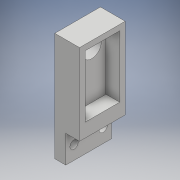
# Autodesk Inventor part: armpart2
Saved by Autodesk Inventor 2018.3 (Build 223284000, 284)
## iProperties
Created: 2019-11-01
Part Number: armpart2
Material: 一般
Document SubType Name: Modeling
Designer: Eiji Nishizawa
Density: 1 g/cm^3
Appearance: 既定
Mass: 3.44311 g
Surface Area: 26.3012 cm^2
Volume: 3.44311 cm^3
Author: Eiji Nishizawa
Autodesk Inventor part; units mm, degrees
ref_plane "YZ Plane" through (0, 0, 0) normal (1, 0, 0) x (0, 1, 0)
ref_plane "XZ Plane" through (0, 0, 0) normal (0, 1, 0) x (-1, 0, 0)
ref_plane "XY Plane" through (0, 0, 0) normal (0, 0, 1) x (1, 0, 0)
sketch "スケッチ1" plane through (0, 0, 0) normal (1, 0, 0) x (0, 1, 0)
  line L0 (8.6678, 22.4898) -> (-7.9322, 22.4898)
  line L1 (-7.9322, 22.4898) -> (-7.9322, -15.0102)
  line L2 (-7.9322, -15.0102) -> (8.6678, -15.0102)
  line L3 (8.6678, -15.0102) -> (8.6678, 22.4898)
  line L4 (8.6678, 22.4898) -> (6.6678, 22.4898)
  line L5 (6.6678, 22.4898) -> (6.6678, -0.0102)
  line L6 (6.6678, -0.0102) -> (8.6678, -0.0102)
  line L7 (8.6678, -0.0102) -> (8.6678, 22.4898)
  line L8 (-7.9322, 22.4898) -> (-5.9322, 22.4898)
  line L9 (-5.9322, 22.4898) -> (-5.9322, -0.0102)
  line L10 (-5.9322, -0.0102) -> (-7.9322, -0.0102)
  line L11 (-7.9322, -0.0102) -> (-7.9322, 22.4898)
  line L12 (8.6678, 22.4898) -> (-7.9322, 22.4898)
  line L13 (-7.9322, 22.4898) -> (-7.9322, 24.4898)
  line L14 (-7.9322, 24.4898) -> (8.6678, 24.4898)
  line L15 (8.6678, 24.4898) -> (8.6678, 22.4898)
  circle A0 centre (5.6678, -10.0102) radius 1.5
  circle A1 centre (-4.9322, -10.0102) radius 1.5
  point P0 (0, 0)
  dimension "d1" = 2
  dimension "d2" = 2
  dimension "d3" = 15
  dimension "d4" = 22.5
  dimension "d5" = 2
  dimension "d6" = 3
  dimension "d7" = 3
  dimension "d8" = 5
  dimension "d9" = 5
  dimension "d10" = 3
  dimension "d11" = 3
  dimension "d25" = 12.6
  dimension "d26" = 16.6
  constraints: 32 end point, 8 parallel, 4 horizontal, 4 perpendicular, 2 centre point, 1 point on line
  measures "d1" distance between parallel lines of L3 L5
  measures "d2" distance between parallel lines of L1 L9
  measures "d3" distance between parallel lines of L6 L2
  measures "d4" distance between parallel lines of L0 L6
  measures "d5" distance between parallel lines of L0 L14
  measures "d6" distance from line of L3 A0.centre
  measures "d7" distance from line of L1 A1.centre
  measures "d8" distance from line of L2 A1.centre
  measures "d9" distance from line of L2 A0.centre
  measures "d10" diameter of A0
  measures "d11" diameter of A1
  measures "d25" distance between parallel lines of L5 L9
  measures "d26" distance between parallel lines of L3 L1
extrude "押し出し1" add sketch "スケッチ1" against normal blind 4
extrude "押し出し2" add sketch "スケッチ1" along normal blind 5 contours L3 L6 L5 L0 | L0 L13 L14 L15 | L9 L10 L1 L0
sketch "スケッチ2" plane through (0, 0, 0) normal (1, 0, 0) x (0, 0, -1)
  circle A0 centre (-17.2898, 1.4678) radius 3.5
  line L0 (-24.4898, 8.6678) -> (-24.4898, -7.9322) projected
  line L1 (0.0102, 8.6678) -> (-24.4898, 8.6678) projected
  line L2 (-24.4898, -7.9322) -> (0.0102, -7.9322) projected
  point P0 (0, 0)
  dimension "d16" = 7
  dimension "d17" = 7.2
  dimension "d18" = 7.2
  dimension "d19" = 9.4
  constraints: 1 centre point
  measures "d16" diameter of A0
  measures "d17" distance from line of L0 A0.centre
  measures "d18" distance from line of L1 A0.centre
  measures "d19" distance from line of A0.centre L2
extrude "押し出し3" cut sketch "スケッチ2" against normal blind 5
sketch "スケッチ3" plane through (0, 0, 0) normal (1, 0, 0) x (0, 0, -1)
  line L0 (-24.4898, 8.6678) -> (15.0102, 8.6678) projected
  line L1 (0.0102, -7.9322) -> (15.0102, -7.9322) projected
  line L2 (0, 8.6678) -> (5, 8.6678)
  line L3 (5, 8.6678) -> (5, -7.9322)
  line L4 (5, -7.9322) -> (0, -7.9322)
  line L5 (0, -7.9322) -> (0, 8.6678)
  point P0 (0, 0)
  dimension "d22" = 5
  constraints: 8 end point, 2 parallel, 2 point on line, 1 horizontal, 1 perpendicular
  measures "d22" distance between parallel lines of L5 L3
extrude "押し出し4" add sketch "スケッチ3" along normal blind 5
